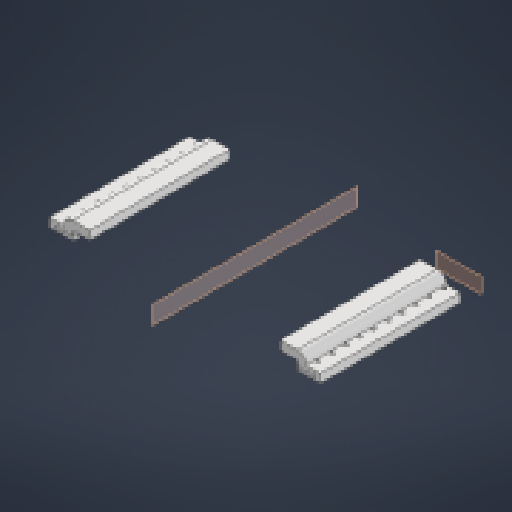
# Autodesk Inventor part: Tourniquet_Rail_01_V3
Saved by Autodesk Inventor 2026.2 (Build 302298000, 298)
## iProperties
Created: 2026-03-04
Part Number: Tourniquet_Rail_01_V3
Material: Generic
Document SubType Name: Modeling
Designer: vckot
Density: 1 g/cm^3
Appearance: Default
Author: vckot
Autodesk Inventor part; units mm, degrees
ref_plane "YZ Plane" through (0, 0, 0) normal (1, 0, 0) x (0, 1, 0)
ref_plane "XZ Plane" through (0, 0, 0) normal (0, 1, 0) x (-1, 0, 0)
ref_plane "XY Plane" through (0, 0, 0) normal (0, 0, 1) x (1, 0, 0)
sketch "Sketch1" plane through (0, 0, 0) normal (0, 1, 0) x (-1, 0, 0)
  line L0 (-6.25, 51.25) -> (6.25, 51.25)
  line L1 (6.25, 51.25) -> (6.25, -51.25)
  line L2 (6.25, -51.25) -> (-6.25, -51.25)
  line L3 (-6.25, -51.25) -> (-6.25, 51.25)
  line L4 (-6.25, 51.25) -> (6.25, -51.25) construction
  line L5 (6.25, 51.25) -> (-6.25, -51.25) construction
  point P0 (0, 0)
  dimension "d0" = 12.5
  dimension "d1" = 102.5
  constraints: 12 end point, 2 midpoint, 2 parallel, 1 horizontal, 1 perpendicular
  measures "d0" distance of L1.end L2.end
  measures "d1" distance of L0.end L1.end
extrude "Extrusion1" add sketch "Sketch1" along normal blind 4.8
sketch "Sketch2" plane through (-6.25, 0, -51.25) normal (-1, 0, 0) x (0, 0, 1)
  line L0 (0, 0) -> (0, 4.8) projected
  line L1 (102.5, 0) -> (102.5, 4.8) projected
  line L2 (0, 2.3) -> (102.5, 2.3)
  line L3 (102.5, 2.3) -> (102.5, 1.45)
  line L4 (102.5, 1.45) -> (0, 1.45)
  line L5 (0, 1.45) -> (0, 2.3)
  line L6 (0, 4.8) -> (102.5, 4.8) projected
  point P0 (51.25, 0)
  point P1 (102.5, 2.4)
  point P2 (0, 1.45)
  dimension "d4" = 0.85
  dimension "d7" = 2.5
  constraints: 8 end point, 2 parallel, 2 point on line, 1 horizontal, 1 midpoint, 1 perpendicular
  measures "d4" distance between parallel lines of L4 L2
  measures "d7" distance between parallel lines of L6 L2
extrude "Extrusion2" cut sketch "Sketch2" against normal blind 10 contours L0 L2 L1 L4
sketch "Sketch3" plane through (0, 4.8, 0) normal (0, 1, 0) x (1, 0, 0)
  line L0 (-6.25, 51.25) -> (-6.25, -51.25) projected
  line L1 (-6.25, -51.25) -> (-15.25, -51.25)
  line L2 (-15.25, -51.25) -> (-15.25, 51.25)
  line L3 (-15.25, 51.25) -> (-6.25, 51.25)
  line L4 (-6.25, 51.25) -> (-6.25, -51.25)
  line L5 (6.25, 51.25) -> (-6.25, 51.25) projected
  line L6 (-6.25, -51.25) -> (6.25, -51.25) projected
  line L7 (-6.25, 51.25) -> (-1.25, 51.25)
  line L8 (-1.25, 51.25) -> (-1.25, -51.25)
  line L9 (-1.25, -51.25) -> (-6.25, -51.25)
  line L10 (-6.25, -51.25) -> (-6.25, 51.25)
  point P0 (0, 0)
  dimension "d8" = 9
  dimension "d9" = 5
  constraints: 16 end point, 4 parallel, 2 horizontal, 2 perpendicular, 1 collinear, 1 point on line
  measures "d8" distance of L2.end L3.end
  measures "d9" distance of L8.end L9.end
extrude "Extrusion3" add sketch "Sketch3" along normal blind 4.75
fillet "Fillet1" radius 4.75 1 edges at (-1.25, 9.55, 0)
ref_plane "Work Plane1" through (-6.25, 0, -33.75) normal (0, 0, 1) x (1, 0, 0)
sketch "Sketch7" plane through (0, 4.8, 0) normal (0, 1, 0) x (1, 0, 0)
  circle A0 centre (0, -46.25) radius 1
  line L0 (-1.25, -51.25) -> (6.25, -51.25) projected
  line L1 (6.25, -51.25) -> (6.25, 51.25) projected
  circle A1 centre (0, -38.75) radius 1
  circle A2 centre (0, -31.25) radius 1
  circle A3 centre (0, -23.75) radius 1
  circle A4 centre (0, -16.25) radius 1
  circle A5 centre (0, -8.75) radius 1
  circle A6 centre (0, -1.25) radius 1
  circle A7 centre (0, 6.25) radius 1
  circle A8 centre (0, 13.75) radius 1
  circle A9 centre (0, 21.25) radius 1
  circle A10 centre (0, 28.75) radius 1
  circle A11 centre (0, 36.25) radius 1
  circle A12 centre (0, 43.75) radius 1
  point P0 (0, 0)
  dimension "d32" = 2
  dimension "d33" = 5
  dimension "d34" = 6.25
  dimension "d37" = 7.5
  constraints: 13 centre point, 1 vertical, 24 other
  measures "d32" diameter of A0
  measures "d33" distance from line of L0 A0.centre
  measures "d34" distance from line of L1 A0.centre
  measures "d37" distance of A0.centre A1.centre
extrude "Extrusion7" cut sketch "Sketch7" against normal through all
ref_plane "Work Plane2" through (-66.25, 12.3, 50) normal (1, 0, 0) x (0, 0, -1)
mirror "Mirror1" about plane through (-66.25, 12.3, 50) normal (1, 0, 0) of "Extrusion1", "Extrusion3", "Extrusion2", "Extrusion7", "Fillet1"
sketch "Sketch8" plane through (6.25, 0, 51.25) normal (1, 0, 0) x (0, 0, -1)
  line L0 (102.5, 4.8) -> (102.5, 9.55) projected
  line L1 (102.5, 9.55) -> (0, 9.55) projected
  line L2 (102.5, 4.8) -> (77.5, 4.8)
  line L3 (77.5, 4.8) -> (77.5, 9.55)
  line L4 (77.5, 9.55) -> (102.5, 9.55)
  line L5 (102.5, 9.55) -> (102.5, 4.8)
  point P0 (51.25, 0)
  dimension "d44" = 25
  constraints: 8 end point, 2 parallel, 1 horizontal, 1 perpendicular, 1 point on line
  measures "d44" distance between parallel lines of L0 L3
extrude "Extrusion8" cut sketch "Sketch8" against normal through all
sketch "Sketch9" plane through (0, 4.8, 0) normal (0, 1, 0) x (1, 0, 0)
  line L0 (-1.25, 26.25) -> (-6.25, 26.25) projected
  line L1 (6.25, -51.25) -> (6.25, 51.25) projected
  line L2 (-6.25, 26.25) -> (6.25, 26.25)
  line L3 (6.25, 26.25) -> (6.25, 51.25)
  line L4 (6.25, 51.25) -> (-6.25, 51.25)
  line L5 (-6.25, 51.25) -> (-6.25, 26.25)
  line L6 (-138.75, 51.25) -> (-126.25, 51.25) projected
  line L7 (-138.75, 51.25) -> (-126.25, 51.25)
  line L8 (-126.25, 51.25) -> (-126.25, 26.25)
  line L9 (-126.25, 26.25) -> (-138.75, 26.25)
  line L10 (-138.75, 26.25) -> (-138.75, 51.25)
  circle A0 centre (-132.5, 28.75) radius 1 projected
  circle A1 centre (-132.5, 36.25) radius 1 projected
  circle A2 centre (-132.5, 43.75) radius 1 projected
  circle A3 centre (0, 28.75) radius 1 projected
  circle A4 centre (0, 36.25) radius 1 projected
  circle A5 centre (0, 43.75) radius 1 projected
  point P0 (0, 0)
  point P1 (6.25, 26.25)
  constraints: 16 end point, 4 parallel, 2 horizontal, 2 perpendicular, 1 point on line
extrude "Extrusion9" add sketch "Sketch9" along normal blind 7.5
body "Solid1"
